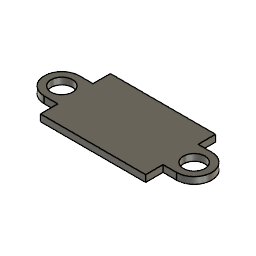
1D_Lidar_CAD (Autodesk Fusion 360 archive; units mm, degrees)
design "test"
Autodesk Fusion 360 part; units mm, degrees
sketch "Sketch1" plane through (0, 0, 0) normal (0, 0, 1) x (1, 0, 0)
  line L0 (0, 0) -> (15.55, 0)
  line L1 (15.55, 0) -> (15.55, 10.34)
  line L2 (15.55, 10.34) -> (0, 10.34)
  line L3 (0, 10.34) -> (0, 0)
  line L4 (15.55, 5.17) -> (15.96, 5.17)
  line L5 (0, 5.17) -> (-0.41, 5.17)
  line L6 (15.96, 5.17) -> (17.55, 5.17)
  circle A0 centre (17.55, 5.17) radius 1.59
  line L7 (-0.41, 5.17) -> (-2, 5.17)
  circle A1 centre (-2, 5.17) radius 1.59
  circle A2 centre (-2, 5.17) radius 2.6
  circle A3 centre (17.55, 5.17) radius 2.6
  line L8 (17.55, 7.77) -> (14.1977, 7.77)
  line L9 (14.1977, 7.77) -> (14.1977, 2.57)
  line L10 (14.1977, 2.57) -> (17.55, 2.57)
  line L11 (17.55, 2.57) -> (17.55, 7.77)
  line L12 (-2.0152, 7.77) -> (2.0676, 7.77)
  line L13 (2.0676, 7.77) -> (2.0676, 2.57)
  line L14 (2.0676, 2.57) -> (-2.0152, 2.57)
  line L15 (-2.0152, 2.57) -> (-2.0152, 7.77)
  dimension "d1" = 15.55
  dimension "d2" = 10.34
  dimension "d3" = 0.41
  dimension "d4" = 0.41
  dimension "d5" = 1.59
  dimension "d6" = 3.18
  dimension "d7" = 1.59
  dimension "d8" = 3.18
  dimension "d9" = 5.2
  dimension "d10" = 5.2
  dimension "d11" = 5.2
  dimension "d12" = 5.2
  constraint horizontal L0
  constraint vertical L1
  constraint horizontal L2
  constraint vertical L3
  constraint coincident L0.start L3.end
  constraint midpoint L1 L4.start
  constraint perpendicular L1 L4
  constraint midpoint L3 L5.start
  constraint perpendicular L3 L5
  constraint perpendicular L1 L6
  constraint coincident L6.end A0.centre
  constraint parallel L5 L7
  constraint coincident L7.end A1.centre
  constraint concentric A1 A2
  constraint concentric A0 A3
  constraint horizontal L8
  constraint vertical L9
  constraint horizontal L10
  constraint vertical L11
  constraint coincident A3 L8.start
  constraint horizontal L12
  constraint vertical L13
  constraint horizontal L14
  constraint vertical L15
  constraint coincident A2 L12.start
  measures "d1" distance of L0.start L0.end
  measures "d2" distance of L0.start L2.end
  measures "d3" distance of L4.start L4.end
  measures "d4" distance of L5.start L5.end
  measures "d5" distance of L4.end L6.end
  measures "d6" diameter of A0
  measures "d7" distance of L5.end L7.end
  measures "d8" diameter of A1
  measures "d9" diameter of A2
  measures "d10" diameter of A3
  measures "d11" distance of L8.start L10.end
  measures "d12" distance of L12.start L14.end
extrude "Extrude1" add sketch "Sketch1" along normal blind 12 contours L0 L1 L2 L3 L8 L9 L10 L12 L13 L14 | L3 A2 L12 | L3 A2 L14 | L3 A2 L12 L13 L14 | L1 A3 L8 L9 L10 | L1 A3 L10 | L3 L5 A1 A2 L15 | L3 A2 | A1 A2 L15 | L1 A3 | L1 L4 A0 A3 L11 | A0 A3 L11 | L3 L5 A1 A2 L15 | L1 L4 A0 A3 L11 | L1 A3 L8
extrude "Extrude2" cut 1 faces at (10.3667, 4.3033, 12) along direction (0, 0, -1) blind 11
shell "Shell1" [rolled back] inner thickness 0.5
equation "d3 = ( ( 16.37 - 15.55 ) / 2 ) * 1 mm"
equation "d5 = ( 3.18 / 2 ) * 1 mm"
equation "d7 = ( 3.18 / 2 ) * 1 mm"

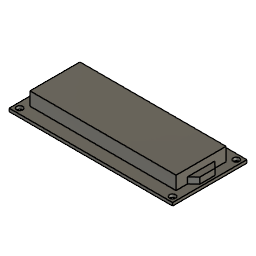
design "Untitled"
Autodesk Fusion 360 part; units mm, degrees
sketch "Sketch1" plane through (0, 0, 0) normal (0, 0, 1) x (1, 0, 0)
  line L0 (0, 0) -> (71.5, 0)
  line L1 (71.5, 0) -> (71.5, 24.5)
  line L2 (71.5, 24.5) -> (0, 24.5)
  line L3 (0, 24.5) -> (0, 0)
  dimension "d1" = 71.5
  dimension "d2" = 24.5
  constraint horizontal L0
  constraint vertical L1
  constraint horizontal L2
  constraint vertical L3
  constraint coincident L0.start L3.end
  measures "d1" distance of L0.start L0.end
  measures "d2" distance of L0.start L2.end
extrude "Extrude1" add sketch "Sketch1" along normal blind 3.5
sketch "Sketch2" plane through (0, 0, 3.5) normal (0, 0, 1) x (-1, 0, 0)
  line L0 (0, -24.5) -> (0, 0)
  line L1 (0, 0) -> (-71.5, 0)
  line L2 (-71.5, 0) -> (-71.5, -24.5)
  line L3 (-71.5, -24.5) -> (0, -24.5)
  line L4 (0, -24.5) -> (-71.5, -24.5)
  line L5 (-71.5, -24.5) -> (-71.5, 0)
  line L6 (-71.5, 0) -> (0, 0)
  line L7 (0, 0) -> (0, -24.5)
  line L8 (0, -12.25) -> (0, -18.92)
  line L9 (0, -12.25) -> (3.11, -12.25)
  line L10 (3.11, -12.25) -> (3.11, -15.965)
  line L11 (3.11, -15.965) -> (0, -18.92)
  line L12 (0, -12.25) -> (0, -5.58)
  line L13 (3.11, -12.25) -> (3.11, -8.535)
  line L14 (3.11, -8.535) -> (0, -5.58)
  line L15 (-35.75, -24.5) -> (-35.75, 0)
  line L16 (-74.61, -15.965) -> (-71.5, -18.92)
  line L17 (-74.61, -12.25) -> (-74.61, -15.965)
  line L18 (-74.61, -12.25) -> (-74.61, -8.535)
  line L19 (-74.61, -8.535) -> (-71.5, -5.58)
  dimension "d5" = 6.67
  dimension "d6" = 3.11
  dimension "d7" = 3.715
  constraint horizontal L4
  constraint vertical L5
  constraint horizontal L6
  constraint vertical L7
  constraint coincident L1.end L2.start
  constraint coincident L0.start L3.end
  constraint midpoint L7 L8.start
  constraint perpendicular L4 L8
  constraint perpendicular L8 L9
  constraint perpendicular L9 L10
  constraint symmetric L8.start L9 L12.start
  constraint symmetric L8.end L9 L12.end
  constraint symmetric L10.start L9 L13.start
  constraint symmetric L9 L10.end L13.end
  constraint midpoint L4 L15.start
  constraint midpoint L6 L15.end
  constraint symmetric L8.end L15 L16.end
  constraint symmetric L9.end L15 L17.start
  constraint symmetric L10.end L15 L16.start
  constraint symmetric L12.end L15 L19.end
  constraint symmetric L13.end L15 L18.end
  measures "d5" distance of L8.start L8.end
  measures "d6" distance of L8.start L9.end
  measures "d7" distance of L9.end L10.end
extrude "Extrude2" add sketch "Sketch2" along normal blind 3
sketch "Sketch3" plane through (0, 0, 6.5) normal (0, 0, 1) x (-1, 0, 0)
  line L0 (-74.61, -8.535) -> (-74.61, -15.965)
  line L1 (-74.61, -15.965) -> (-71.5, -18.92)
  line L2 (-71.5, -18.92) -> (-71.5, -24.5)
  line L3 (-71.5, -24.5) -> (0, -24.5)
  line L4 (0, -24.5) -> (0, -18.92)
  line L5 (0, -18.92) -> (3.11, -15.965)
  line L6 (3.11, -15.965) -> (3.11, -8.535)
  line L7 (3.11, -8.535) -> (0, -5.58)
  line L8 (0, -5.58) -> (0, 0)
  line L9 (0, 0) -> (-71.5, 0)
  line L10 (-71.5, 0) -> (-71.5, -5.58)
  line L11 (-71.5, -5.58) -> (-74.61, -8.535)
  line L12 (-35.75, -24.5) -> (-35.75, 0)
  line L13 (3.11, -12.25) -> (-74.61, -12.25)
  line L14 (-35.75, -12.25) -> (-75.75, -12.25)
  line L15 (-75.75, -12.25) -> (-75.75, -30.435)
  line L16 (-75.75, -30.435) -> (-35.75, -30.435)
  line L17 (-35.75, -30.435) -> (-35.75, -12.25)
  line L18 (4.25, -30.435) -> (-35.75, -30.435)
  line L19 (4.25, -12.25) -> (4.25, -30.435)
  line L20 (-74.61, -12.25) -> (3.11, -12.25)
  line L21 (-35.75, -12.25) -> (4.25, -12.25)
  line L22 (4.25, 5.935) -> (-35.75, 5.935)
  line L23 (4.25, -12.25) -> (4.25, 5.935)
  line L24 (-75.75, 5.935) -> (-35.75, 5.935)
  line L25 (-75.75, -12.25) -> (-75.75, 5.935)
  dimension "d10" = 40
  dimension "d11" = 18.185
  constraint midpoint L3 L12.start
  constraint midpoint L9 L12.end
  constraint midpoint L6 L13.start
  constraint midpoint L0 L13.end
  constraint horizontal L14
  constraint vertical L15
  constraint horizontal L16
  constraint vertical L17
  constraint midpoint L12 L14.start
  constraint symmetric L12 L13.start L13.end
  constraint symmetric L12 L13.end L13.start
  constraint symmetric L12 L14.start L17.end
  constraint symmetric L12 L14.end L19.start
  constraint symmetric L12 L15.end L18.start
  constraint symmetric L12 L16.end L17.start
  constraint symmetric L13 L14.end L15.start
  constraint symmetric L13 L15.end L24.start
  constraint symmetric L13 L16.end L22.end
  constraint symmetric L13 L18.start L22.start
  constraint symmetric L13 L19.start L21.end
  measures "d10" distance of L14.start L14.end
  measures "d11" distance of L14.start L16.end
extrude "Extrude3" add sketch "Sketch3" along normal blind 1.5
move_body "Move1" bodies 1 to x (1, 0, 0) y (0, -1, 0) z (0, 0, -1) at (0, -11.87, 0)
move_body "Move3" bodies 1 to x (1, 0, 0) y (0, 1, 0) z (0, 0, 1) at (0, 24, 8)
hole "Hole1" at (-1.65, 15.465, 1.5) direction (0, 0, -1) diameter 3 depth 1.5 tip angle 118
hole "Hole2" at (73.15, 15.465, 1.5) direction (0, 0, -1) diameter 3 depth 1.5 tip angle 118
hole "Hole3" at (-1.65, -15.705, 1.5) direction (0, 0, -1) diameter 3 depth 1.5 tip angle 118
hole "Hole4" at (73.15, -15.705, 1.5) direction (0, 0, -1) diameter 3 depth 1.5 tip angle 118
move_body "Move2" [suppressed]
equation "d5 = ( 13.34 / 2 ) * 1 mm"
equation "d7 = ( 7.43 / 2 ) * 1 mm"
equation "d11 = ( 36.37 / 2 ) * 1 mm"
